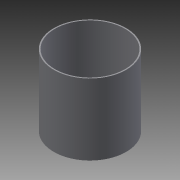
# Autodesk Inventor part: Detection Region Vacuum Collar
Saved by Autodesk Inventor 2014 (Build 180170000, 170)
## iProperties
Created: 2014-05-16
Part Number: Detection Region Vacuum Collar
Material: Generic
Document SubType Name: Modeling
Designer: ijs09
Density: 1 g/cm^3
Appearance: Default
GlobalPropertyList: <PropertyList/>
Author: ijs09
Autodesk Inventor part; units mm, degrees
ref_plane "YZ Plane" through (0, 0, 0) normal (1, 0, 0) x (0, 1, 0)
ref_plane "XZ Plane" through (0, 0, 0) normal (0, 1, 0) x (-1, 0, 0)
ref_plane "XY Plane" through (0, 0, 0) normal (0, 0, 1) x (1, 0, 0)
sketch "Sketch1" plane through (0, 0, 0) normal (0, 0, 1) x (1, 0, 0)
  circle A0 centre (0, 0) radius 98.552
  circle A1 centre (0, 0) radius 101.85
  dimension "d0" = 197.104
  dimension "d1" = 203.7
  constraints: 2 centre point, 2 coincident
  measures "d0" diameter of A0
  measures "d1" diameter of A1
extrude "Extrusion1" add sketch "Sketch1" along normal blind 200
body "Solid1"
